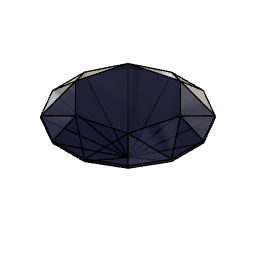
diamond (Autodesk Fusion 360 design; units mm, degrees)
Autodesk Fusion 360 part; units mm, degrees
sketch "Sketch1" plane through (0, 0, 0) normal (0, 0, 1) x (1, 0, 0)
  line L0 (-13.3975, 50) -> (-36.6025, 36.6025)
  line L1 (-36.6025, 36.6025) -> (-50, 13.3975)
  line L2 (-50, 13.3975) -> (-50, -13.3975)
  line L3 (-50, -13.3975) -> (-36.6025, -36.6025)
  line L4 (-36.6025, -36.6025) -> (-13.3975, -50)
  line L5 (-13.3975, -50) -> (13.3975, -50)
  line L6 (13.3975, -50) -> (36.6025, -36.6025)
  line L7 (36.6025, -36.6025) -> (50, -13.3975)
  line L8 (50, -13.3975) -> (50, 13.3975)
  line L9 (50, 13.3975) -> (36.6025, 36.6025)
  line L10 (36.6025, 36.6025) -> (13.3975, 50)
  line L11 (13.3975, 50) -> (-13.3975, 50)
  dimension "d1" = 50
  measures "d1" distance of origin L11
extrude "Extrude1" add sketch "Sketch1" against normal blind 34 draft -60
extrude "Extrude2" add 1 faces at (16.6667, -4.4658, 0) along direction (0, 0, 1) blind 1.5 draft -5
extrude "Extrude3" add 1 faces at (0, 8.9082, 1.5) along direction (0, 0, 1) blind 12.5 draft -50.5
ref_plane "WorkPlane1" through (25.4059, -25.4059, 14) normal (-0.542071, 0.145248, -0.827685) x (-0.258819, -0.965926, 0)
sketch "Sketch2" plane through (25.4059, -25.4059, 14) normal (-0.542071, 0.145248, -0.827685) x (-0.258819, -0.965926, 0)
  line L0 (0, 0) -> (-35.9293, 0)
  line L1 (-35.9293, 0, 0) -> (-17.9647, -23.9926, -1.1653)
  line L2 (-17.9647, -23.9926, -1.1653) -> (0, 0, 0)
  point P0 (-35.9293, 0)
  point P1 (-17.9647, -23.9926)
  constraint coincident L0.start origin
  constraint coincident P0 L0.end
extrude "Extrude4" cut sketch "Sketch2" against normal blind 17 contours L0 L1 L2 in plane through (25.4059, -25.4059, 14) normal (-0.502649, 0.134684, -0.853934)
pattern_circular "C-Pattern1" count 6 over 360 about axis through (0, 0, 1.75) along (0, 0, 1) of "Extrude4"
